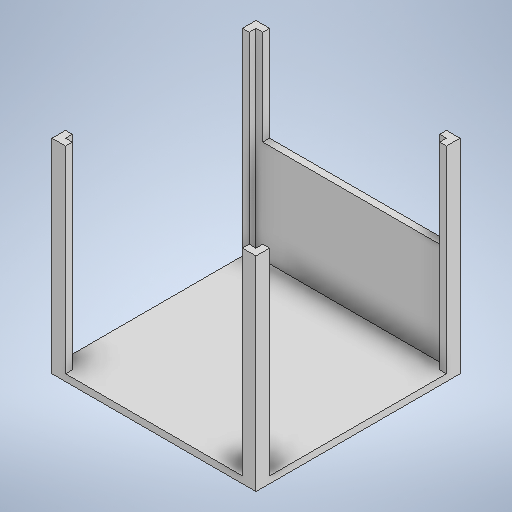
# Autodesk Inventor part: 적재부 하판
Saved by Autodesk Inventor 2025 (Build 290162000, 162)
## iProperties
Created: 2024-06-08
Part Number: 적재부 하판
Material: 일반
Document SubType Name: Modeling
Designer: goomi
Density: 1 g/cm^3
Appearance: 기본값
Author: goomi
Autodesk Inventor part; units mm, degrees
ref_plane "YZ Plane" through (0, 0, 0) normal (1, 0, 0) x (0, 1, 0)
ref_plane "XZ Plane" through (0, 0, 0) normal (0, 1, 0) x (-1, 0, 0)
ref_plane "XY Plane" through (0, 0, 0) normal (0, 0, 1) x (1, 0, 0)
sketch "스케치1" plane through (0, 0, 0) normal (0, 0, 1) x (1, 0, 0)
  line L0 (0, 0) -> (150, 0)
  line L1 (150, 0) -> (150, 150)
  line L2 (0, 150) -> (0, 0)
  line L3 (0, 80) -> (150, 80)
  line L4 (0, 5) -> (150, 5)
  line L5 (0, 150) -> (10, 150)
  line L6 (10, 150) -> (10, 80)
  line L7 (10, 80) -> (0, 80)
  line L8 (0, 80) -> (0, 150)
  line L9 (150, 150) -> (140, 150)
  line L10 (140, 150) -> (140, 80)
  line L11 (140, 80) -> (150, 80)
  line L12 (150, 80) -> (150, 150)
  line L13 (150, 150) -> (140, 150)
  line L14 (10, 150) -> (0, 150)
  dimension "d0" = 150
  dimension "d1" = 150
  dimension "d2" = 80
  dimension "d3" = 5
  dimension "d4" = 10
  dimension "d5" = 10
  constraints: 30 end point, 7 parallel, 6 point on line, 4 horizontal, 4 perpendicular
  measures "d0" distance of L2.start L1.end
  measures "d1" distance of L1.end L0.end
  measures "d2" distance between parallel lines of L0 L3
  measures "d3" distance between parallel lines of L0 L4
  measures "d4" distance of L6.end L7.end
  measures "d5" distance of L11.end L10.end
extrude "돌출1" add sketch "스케치1" along normal blind 150 contours L2 L4 L1 L0
extrude "돌출2" add sketch "스케치1" along normal blind 5 contours L2 L3 L1 L4
extrude "돌출3" add sketch "스케치1" along normal blind 5 contours L2 L5 L6 L3 | L3 L10 L9 L1
sketch "스케치2" plane through (0, 5, 150) normal (0, 1, 0) x (1, 0, 0)
  line L0 (150, 145) -> (0, 145) projected
  line L1 (0, 145) -> (0, 0) projected
  line L2 (150, 0) -> (0, 0) projected
  line L3 (150, 145) -> (150, 0) projected
  line L4 (140, 145) -> (140, 150) projected
  line L5 (140, 150) -> (10, 150) projected
  line L6 (10, 150) -> (10, 145) projected
  line L7 (140, 145) -> (10, 145) projected
  line L8 (10, 150) -> (0, 150) projected
  line L9 (0, 150) -> (0, 145) projected
  line L10 (10, 145) -> (0, 145) projected
  line L11 (10, 150) -> (10, 145) projected
  line L12 (150, 150) -> (140, 150) projected
  line L13 (140, 150) -> (140, 145) projected
  line L14 (150, 145) -> (140, 145) projected
  line L15 (150, 150) -> (150, 145) projected
  line L16 (0, 150) -> (5, 150)
  line L17 (5, 150) -> (5, 140)
  line L18 (5, 140) -> (0, 140)
  line L19 (0, 140) -> (0, 150)
  line L20 (0, 150) -> (150, 150) projected
  line L21 (0, 150) -> (0, 140)
  line L22 (5, 140) -> (5, 145)
  line L23 (10, 145) -> (10, 150)
  line L24 (0, 75) -> (150, 75)
  line L25 (150, 145) -> (150, 0) projected
  line L26 (75, 0) -> (75, 150)
  line L27 (10, 0) -> (10, 5)
  line L28 (10, 0) -> (0, 0)
  line L29 (5, 5) -> (5, 10)
  line L30 (5, 10) -> (0, 10)
  line L31 (0, 10) -> (0, 0)
  line L32 (5, 5) -> (10, 5)
  line L33 (5, 145) -> (10, 145)
  line L34 (10, 150.1761) -> (0, 150)
  line L35 (10, 0) -> (0, 0)
  line L36 (0, 145) -> (150, 145)
  line L37 (150, 145) -> (150, 0)
  line L38 (0, 0) -> (150, 0)
  line L39 (140, 150) -> (140, 145)
  line L40 (145, 140) -> (150, 140)
  line L41 (145, 140) -> (145, 145)
  line L42 (145, 10) -> (150, 10)
  line L43 (150, 10) -> (150, 0)
  line L44 (145, 5) -> (145, 10)
  line L45 (145, 5) -> (140, 5)
  line L46 (140, 0) -> (140, 5)
  point P0 (5, 0)
  point P1 (140, 5)
  point P2 (140, 0)
  point P3 (150, 10)
  point P4 (0, 10)
  point P5 (0, 140)
  dimension "d12" = 5
  dimension "d13" = 10
  dimension "d14" = 150
  dimension "d15" = 10
  dimension "d16" = 150
  dimension "d17" = 150
  constraints: 58 end point, 25 symmetric about line, 2 collinear, 2 horizontal, 2 midpoint, 2 parallel, 2 perpendicular, 2 point on line, 1 vertical, 2 other
  measures "d12" distance of L17.end L18.end
  measures "d13" distance of L16.end L17.end
  measures "d14" distance of L1.end L8.end
  measures "d15" distance of L21.start L18.end
  measures "d16" distance of L12.start L21.start
  measures "d17" diameter of L2 L24
extrude "돌출4" add sketch "스케치2" along normal blind 145 contours L3 L40 L41 L0 | L3 L2 L46 L45 L44 L42 | L17 L18 L1 L0 | L30 L29 L32 L27 L2 L1
